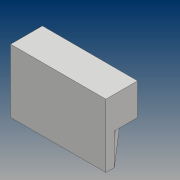
# Autodesk Inventor part: 41 (61598.433 mm^3)
Saved by Autodesk Inventor 2018 (Build 220112000, 112)
## iProperties
Created: 2020-09-18
Part Number: 41 (61598.433 mm^3)
Material: 一般
Document SubType Name: Modeling
Designer: 88697
Density: 1 g/cm^3
Appearance: 預設
Author: 88697
Autodesk Inventor part; units mm, degrees
ref_plane "YZ Plane" through (0, 0, 0) normal (1, 0, 0) x (0, 1, 0)
ref_plane "XZ Plane" through (0, 0, 0) normal (0, 1, 0) x (-1, 0, 0)
ref_plane "XY Plane" through (0, 0, 0) normal (0, 0, 1) x (1, 0, 0)
sketch "草圖1" plane through (0, 0, 0) normal (1, 0, 0) x (0, 1, 0)
  line L0 (0, 0) -> (20, 0)
  line L1 (20, 0) -> (20, -20)
  line L2 (20, -20) -> (0, -20)
  line L3 (0, -20) -> (0, 0)
  line L4 (0, 0) -> (5.3281, 0)
  line L5 (5.3281, 0) -> (5.3281, -40)
  line L6 (5.3281, -40) -> (0, -40)
  line L7 (0, -40) -> (0, 0)
  dimension "d0" = 40
  dimension "d1" = 20
  dimension "d2" = 20
  constraints: 16 end point, 4 parallel, 2 horizontal, 2 perpendicular
  measures "d0" distance of L6.end L0.start
  measures "d1" distance between parallel lines of L3 L1
  measures "d2" distance of L0.end L1.end
extrude "擠出1" add sketch "草圖1" along normal blind 60
sketch "草圖2" plane through (0, 0, -40) normal (0, 0, -1) x (-1, 0, 0)
  line L0 (0, 0) -> (0, 5.3281) projected
  line L1 (0, 0) -> (0, 40)
  line L2 (0, 40) -> (-30, 40)
  line L3 (0, 5.3281) -> (-60, 5.3281) projected
  line L4 (-30, 40) -> (-60, 5.3281)
  line L5 (-60, 5.3281) -> (-60, 0)
  line L6 (0, 0) -> (-60, 0) projected
  line L7 (-60, 0) -> (0, 0)
  dimension "d5" = 30
  dimension "d6" = 40
  constraints: 10 end point, 1 collinear, 1 parallel, 1 perpendicular, 1 vertical
  measures "d5" distance of L1.end L2.end
  measures "d6" distance between parallel lines of L6 L2
extrude "擠出2" add sketch "草圖2" against normal up to surface (20 mm away) contours L3 L4 L2 L1
